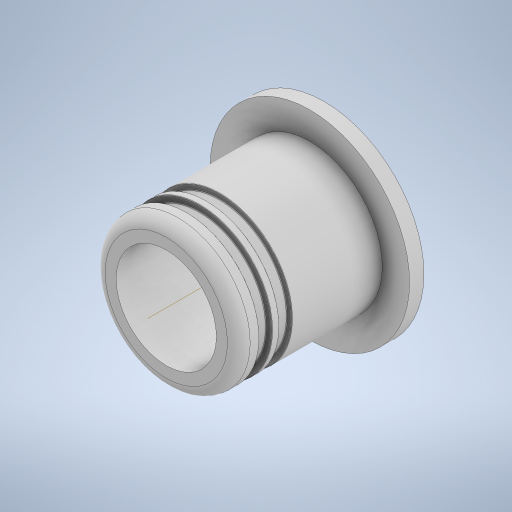
# Autodesk Inventor part: PVCTop2
Saved by Autodesk Inventor 2024 (Build 280153000, 153)
## iProperties
Created: 2024-10-24
Part Number: PVCTop2
Material: Generic
Document SubType Name: Modeling
Designer: bfs7357
Density: 1 g/cm^3
Appearance: Default
Author: bfs7357
Autodesk Inventor part; units mm, degrees
note: some values were not read from the file. Chosen so that the rebuilt part matches the saved one: second side of "Extrusion2".
ref_plane "YZ Plane" through (0, 0, 0) normal (1, 0, 0) x (0, 1, 0)
ref_plane "XZ Plane" through (0, 0, 0) normal (0, 1, 0) x (-1, 0, 0)
ref_plane "XY Plane" through (0, 0, 0) normal (0, 0, 1) x (1, 0, 0)
sketch "Sketch1" plane through (0, 0, 0) normal (0, 0, 1) x (1, 0, 0)
  circle A0 centre (0, 0) radius 27.813
  dimension "d0" = 55.626
  constraints: 1 centre point, 1 coincident
  measures "d0" diameter of A0
extrude "Extrusion1" add sketch "Sketch1" along normal blind 4
sketch "Sketch2" plane through (0, 0, 4) normal (0, 0, 1) x (1, 0, 0)
  circle A0 centre (0, 0) radius 20.2057
  dimension "d3" = 40.4114
  constraints: 1 centre point, 1 coincident
  measures "d3" diameter of A0
extrude "Extrusion2" add sketch "Sketch2" along normal blind 40
sketch "Sketch5" plane through (0, 0, 0) normal (0, 0, -1) x (-1, 0, 0)
  circle A0 centre (0, 0) radius 3.5052
  dimension "d14" = 7.0104
  constraints: 1 centre point, 1 coincident
  measures "d14" diameter of A0
extrude "Extrusion5" cut sketch "Sketch5" against normal blind 16.256
thread "Thread1" size "M16x1.5" class "6H" standard "ISO Metric profile" length 4
sketch "Sketch7" plane through (0, 0, 0) normal (1, 0, 0) x (0, 1, 0)
  line L0 (20.2057, 44) -> (-20.2057, 44) projected
  line L1 (-20.2057, 4) -> (-20.2057, 44) projected
  line L2 (20.4597, 29.172) -> (20.4597, 32.728)
  line L3 (18.9865, 29.172) -> (20.4597, 29.172)
  line L4 (20.4597, 32.728) -> (18.9865, 32.728)
  line L5 (18.8087, 32.5502) -> (18.8087, 29.3498)
  arc A0 (18.9865, 32.728) -> (18.8087, 32.5502) centre (18.9865, 32.5502) ccw
  arc A1 (18.8087, 29.3498) -> (18.9865, 29.172) centre (18.9865, 29.3498) ccw
  line L6 (0, -8.8) -> (0, 52.8) projected
  point P0 (0, 0)
  point P1 (18.8087, 29.172)
  dimension "d28" = 1.651
  dimension "d29" = 0.1778
  constraints: 8 end point, 4 point on circle, 4 tangent, 2 centre point, 2 perpendicular, 2 point on line, 1 equal radius, 1 horizontal
  measures "d28" distance of point (18.809, 29.172) L2.start
  measures "d29" radius of A0
revolve "Revolution1" cut sketch "Sketch7" angle 360 about axis through (0, 0, 4) along (0, 0, 1)
fillet "Fillet1" radius 0.127 1 edges at (-20.2057, 0, 29.172)
fillet "Fillet2" radius 0.127 1 edges at (-20.2057, 0, 32.728)
sketch "Sketch8" plane through (0, 0, 0) normal (1, 0, 0) x (0, 1, 0)
  line L0 (20.2057, 32.855) -> (20.2057, 44) projected
  line L1 (20.2057, 38.278) -> (20.2057, 34.722)
  line L2 (20.2057, 38.278) -> (18.5547, 38.278)
  line L3 (20.2057, 34.722) -> (18.5547, 34.722)
  line L4 (18.5547, 34.722) -> (18.5547, 38.278)
  line L5 (0, -9) -> (0, 54) projected
  point P0 (0, 0)
  point P1 (20.2057, 36.5)
  dimension "d33" = 7.5
  dimension "d34" = 1.778
  dimension "d35" = 1.778
  dimension "d36" = 1.651
  dimension "d37" = 1.651
  constraints: 8 end point, 3 point on line, 2 horizontal
  measures "d33" distance of L0.end point (20.206, 36.5)
  measures "d34" distance of L1.start point (20.206, 36.5)
  measures "d35" distance of L1.end point (20.206, 36.5)
  measures "d36" distance of L1.start L2.end
  measures "d37" distance of L1.end L3.end
revolve "Revolution2" cut sketch "Sketch8" angle 360 about axis through (0, 0, 4) along (0, 0, 1)
fillet "Fillet3" radius 0.1778 2 edges at (0, -18.5547, 34.722) (0, -18.5547, 38.278)
fillet "Fillet4" radius 0.127 2 edges at (-20.2057, 0, 38.278) (-20.2057, 0, 34.722)
sketch "Sketch9" plane through (0, 0, 0) normal (0, 0, -1) x (-1, 0, 0)
  circle A0 centre (0, 0) radius 8.128
  dimension "d41" = 16.256
  constraints: 1 centre point, 1 coincident
  measures "d41" diameter of A0
extrude "Extrusion7" cut sketch "Sketch9" against normal blind 10
fillet "Fillet5" radius 3.175 1 edges at (-20.2057, 0, 44)
sketch "Sketch10" plane through (0, 0, 44) normal (0, 0, 1) x (1, 0, 0)
  circle A0 centre (0, 0) radius 13.97
  dimension "d47" = 27.94
  constraints: 1 centre point, 1 coincident
  measures "d47" diameter of A0
extrude "Extrusion8" cut sketch "Sketch10" against normal blind 40
body "Solid1"
